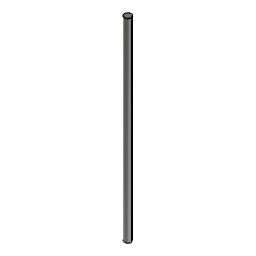
Steering_Shaft Mock v1 (Autodesk Fusion 360 design; units mm, degrees)
Autodesk Fusion 360 part; units mm, degrees
note: some values were not read from the file. Set by a fixed rule: which sketch regions a step uses.
sketch "Sketch1" plane through (0, 0, 0) normal (0, 0, 1) x (1, 0, 0)
  circle A0 centre (0, 0) radius 7.5
  line L0 (2.2175, 7.1647) -> (7.4999, -0.0289)
  dimension "d1" = 15
  constraint coincident A0.centre origin
  constraint coincident A0 L0.start
  constraint coincident A0 L0.end
  measures "d1" diameter of A0
extrude "Extrude1" add sketch "Sketch1" along normal blind 400 contours A0 L0 picked at (-0.1624, -2.0405)
chamfer "Chamfer1" distance 0.5 angle 45 1 faces at (7.461, -0.7641, 133.3333)
sketch "Sketch2" plane through (0, 0, 400) normal (0, 0, 1) x (-1, 0, 0)
  arc A0 (-2.7525, -6.4361) -> (-6.9649, -0.6997) centre (0, 0) ccw
  line L0 (-6.9649, -0.6997) -> (-2.7525, -6.4361)
